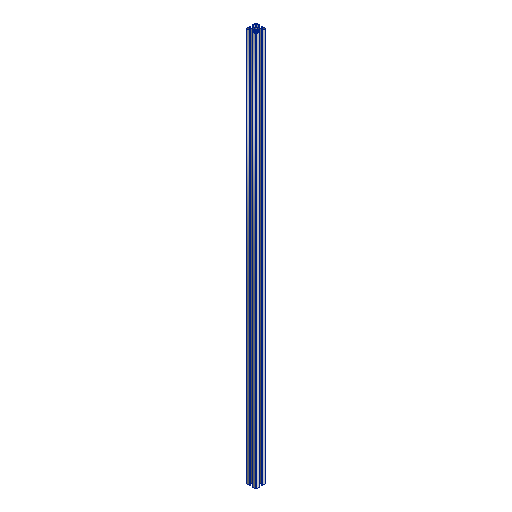
# Autodesk Inventor part: KNFS5-2020
Saved by Autodesk Inventor 2022 (Build 260153000, 153)
## iProperties
Category: PARTsolutions
Company: MISUMI
Part Number: KNFS5-2020
Material: アルミニウム 6061
Catalog Web Link: www.cadenas.de
Description: KHFS5-2020, KHFSB5-2020, KNFS5-2020, KCAF5-2020, KHFSY5-2020-HFS5 Series Aluminum Extrusions 20,25,40mm Square - 1 Slot - Four Slots per - Side - Fixed Length Extrusion
Vendor: MISUMI
Document SubType Name: Modeling
Designer: partserver
Manufacturer: MISUMI
Mass: 725.051 g
Surface Area: 6966.3 cm^2
Volume: 725.051 cm^3
Density: 2.7 g/cm^3
Appearance: アルミニウム - フラット
L: 4000
PSOL_IDENT_0: {$CADENAS_DATA\23d-libs\misumi\metric\38_al_extrusions_blackets\5\khfs5_2020.prj},225 {VTYP=3D},{NB=
PSOL_IDENT_1: KNFS5-2020-4000},{LINA=KNFS5-2020-4000},{NN=KHFS5-2020, KHFSB5-2020, KNFS5-2020, KCAF5-2020, KHFSY5-
PSOL_IDENT_2: 2020},{DATE=08.06.2021 08:25:20},{GEOMDATE=15.11.2016 12:28:43},{VERSION=},{LINEID=570},{WBVAR=},{WB
PSOL_IDENT_3: NUMERIC=}  {NB=KNFS5-2020-4000},{LINA=KNFS5-2020-4000},{KT=1},{PN=KNFS5-2020-4000},{TPS=KNFS5-2020},
PSOL_IDENT_4: {TP=KNFS5},{FRM=2020},{MAT=A6N01SS-T5 Aluminum Alloy or 6005A-T5 Aluminum Alloy},{ST=Black Anodize},
PSOL_IDENT_5: {FEAT=Four-Side Slots},{L=4000},{LTOL=+/- 0.5},{MASS=0},{SA=153},{GMILX=0.57x10^4},{GMILY=0.57x10^4}
PSOL_IDENT_6: ,{CLF=NFS5-2020},{WIDTH=20.000},{HEIGHT=20.000},{VER=6},{DIM=1},{DRILLDIA=4.200},{FRMW=20.000},{FRMH=
PSOL_IDENT_7: 20.000},{FRD=4.200}
NB: KNFS5-2020-4000
NN: KHFS5-2020, KHFSB5-2020, KNFS5-2020, KCAF5-2020, KHFSY5-2020
NT: HFS5 Series Aluminum Extrusions 20,25,40mm Square - 1 Slot - Four Slots per - Side - Fixed Length Extrusion
NBSYN: $PN.
LINA: KNFS5-2020-4000
CATALOG: Misumi
PN: KNFS5-2020-4000
TPS: KNFS5-2020
SUPPLIER: MISUMI
ARTICLENO: KNFS5-2020-4000
BOMINFO: KNFS5-2020-4000
CREATOR: CADENAS GmbH
Title: KNFS5-2020-4000
Author: Cadenas PARTsolutions
Comments: HFS5 Series Aluminum Extrusions 20,25,40mm Square - 1 Slot - Four Slots per - Side - Fixed Length Extrusion
Autodesk Inventor part; units mm, degrees
ref_plane "YZ Plane" through (0, 0, 0) normal (1, 0, 0) x (0, 1, 0)
ref_plane "XZ Plane" through (0, 0, 0) normal (0, 1, 0) x (-1, 0, 0)
ref_plane "XY Plane" through (0, 0, 0) normal (0, 0, 1) x (1, 0, 0)
sketch "_____4" plane through (0, 0, 0) normal (0, 0, 1) x (1, 0, 0)
  line L0 (-10, -3) -> (-10, -9)
  arc A0 (-10, -9) -> (-9, -10) centre (-9, -9) ccw
  line L1 (-9, -10) -> (-3, -10)
  line L2 (-3, -10) -> (-3, -8)
  line L3 (-3, -8) -> (-6, -8)
  line L4 (-6, -8) -> (-6, -7.0607)
  line L5 (-6, -7.0607) -> (-2.9393, -4)
  line L6 (-2.9393, -4) -> (-0.6536, -4)
  arc A1 (-0.6536, -4) -> (-0.4036, -3.933) centre (-0.6536, -3.5) ccw
  line L7 (-0.4036, -3.933) -> (0, -3.7)
  line L8 (0, -3.7) -> (0.4036, -3.933)
  arc A2 (0.4036, -3.933) -> (0.9036, -3.933) centre (0.6536, -3.5) ccw
  line L9 (0.9036, -3.933) -> (1.2189, -3.751)
  line L10 (1.2189, -3.751) -> (2.5, -4)
  line L11 (2.5, -4) -> (2.9393, -4)
  line L12 (2.9393, -4) -> (6, -7.0607)
  line L13 (6, -7.0607) -> (6, -8)
  line L14 (6, -8) -> (3, -8)
  line L15 (3, -8) -> (3, -10)
  line L16 (3, -10) -> (9, -10)
  arc A3 (9, -10) -> (10, -9) centre (9, -9) ccw
  line L17 (10, -9) -> (10, -3)
  line L18 (10, -3) -> (8, -3)
  line L19 (8, -3) -> (8, -6)
  line L20 (8, -6) -> (7.0607, -6)
  line L21 (7.0607, -6) -> (4, -2.9393)
  line L22 (4, -2.9393) -> (4, -0.6536)
  arc A4 (4, -0.6536) -> (3.933, -0.4036) centre (3.5, -0.6536) ccw
  line L23 (3.933, -0.4036) -> (3.7, 0)
  line L24 (3.7, 0) -> (3.933, 0.4036)
  arc A5 (3.933, 0.4036) -> (3.933, 0.9036) centre (3.5, 0.6536) ccw
  line L25 (3.933, 0.9036) -> (3.751, 1.2189)
  line L26 (3.751, 1.2189) -> (4, 2.5)
  line L27 (4, 2.5) -> (4, 2.9393)
  line L28 (4, 2.9393) -> (7.0607, 6)
  line L29 (7.0607, 6) -> (8, 6)
  line L30 (8, 6) -> (8, 3)
  line L31 (8, 3) -> (10, 3)
  line L32 (10, 3) -> (10, 9)
  arc A6 (10, 9) -> (9, 10) centre (9, 9) ccw
  line L33 (9, 10) -> (3, 10)
  line L34 (3, 10) -> (3, 8)
  line L35 (3, 8) -> (6, 8)
  line L36 (6, 8) -> (6, 7.0607)
  line L37 (6, 7.0607) -> (2.9393, 4)
  line L38 (2.9393, 4) -> (0.6536, 4)
  arc A7 (0.6536, 4) -> (0.4036, 3.933) centre (0.6536, 3.5) ccw
  line L39 (0.4036, 3.933) -> (0, 3.7)
  line L40 (0, 3.7) -> (-0.4036, 3.933)
  arc A8 (-0.4036, 3.933) -> (-0.9036, 3.933) centre (-0.6536, 3.5) ccw
  line L41 (-0.9036, 3.933) -> (-1.2189, 3.751)
  line L42 (-1.2189, 3.751) -> (-2.5, 4)
  line L43 (-2.5, 4) -> (-2.9393, 4)
  line L44 (-2.9393, 4) -> (-6, 7.0607)
  line L45 (-6, 7.0607) -> (-6, 8)
  line L46 (-6, 8) -> (-3, 8)
  line L47 (-3, 8) -> (-3, 10)
  line L48 (-3, 10) -> (-9, 10)
  arc A9 (-9, 10) -> (-10, 9) centre (-9, 9) ccw
  line L49 (-10, 9) -> (-10, 3)
  line L50 (-10, 3) -> (-8, 3)
  line L51 (-8, 3) -> (-8, 6)
  line L52 (-8, 6) -> (-7.0607, 6)
  line L53 (-7.0607, 6) -> (-4, 2.9393)
  line L54 (-4, 2.9393) -> (-4, 0.6536)
  arc A10 (-4, 0.6536) -> (-3.933, 0.4036) centre (-3.5, 0.6536) ccw
  line L55 (-3.933, 0.4036) -> (-3.7, 0)
  line L56 (-3.7, 0) -> (-3.933, -0.4036)
  arc A11 (-3.933, -0.4036) -> (-3.933, -0.9036) centre (-3.5, -0.6536) ccw
  line L57 (-3.933, -0.9036) -> (-3.751, -1.2189)
  line L58 (-3.751, -1.2189) -> (-4, -2.5)
  line L59 (-4, -2.5) -> (-4, -2.9393)
  line L60 (-4, -2.9393) -> (-7.0607, -6)
  line L61 (-7.0607, -6) -> (-8, -6)
  line L62 (-8, -6) -> (-8, -3)
  line L63 (-8, -3) -> (-10, -3)
  constraints: 128 end point, 24 point on circle, 12 centre point
extrude "Extrusion1" add sketch "_____4" against normal blind 800
sketch "Sketch2" plane through (0, 0, -800) normal (0, 0, -1) x (-1, 0, 0)
  point P0 (0, 0)
hole "Hole1" at (0, 0, -800) direction (0, 0, 1) diameter 4.2 depth 4000
body "Solid1"
